Autodesk Inventor part; units mm, degrees
(part 2 of 2)
sketch "Sketch3" plane through (9, 0, 0) normal (1, 0, 0) x (0, 0, -1)
  line L0 (-1.5, 0) -> (1.5, 0)
  line L1 (1.5, 0) -> (1.5, 9)
  line L2 (1.5, 9) -> (-1.5, 9)
  line L3 (-1.5, 9) -> (-1.5, 0)
  point P0 (0, 0)
  point P1 (0, 0)
  dimension "d21" = 9
  dimension "d22" = 3
  constraints: 8 end point, 2 parallel, 1 coincident, 1 horizontal, 1 midpoint, 1 perpendicular
  measures "d21" distance of L0.end L1.end
  measures "d22" distance of L0.start L0.end
extrude "Extrusion3" cut sketch "Sketch3" against normal through all
fillet "Fillet2" radius 0.1 12 edges at (4.5, 9, 1.5) (4.5, 9, -1.5) (8.9707, 7.3784, -1.5) (9, 8.2253, -1.5) (4.5, 7.3485, -1.5) (8.9707, 7.3784, 1.5) (9, 8.2253, 1.5) (4.5, 7.3485, 1.5) (9, 9, 0) (0, 9, 0) (0, 8.2253, 1.5) (0, 8.2253, -1.5)
body "Solid1"
